Autodesk Inventor part; units mm, degrees
(part 2 of 2)
sketch "Sketch70" plane through (80, 0, -85) normal (-1, 0, 0) x (0, 0, 1)
  line L0 (155.5, 281.1154) -> (155.5, 497.1154) projected
  line L1 (155.5, 497.1154) -> (14.5, 497.1154) projected
  line L2 (14.5, 497.1154) -> (14.5, 281.1154) projected
  line L3 (14.5, 281.1154) -> (155.5, 281.1154) projected
  line L4 (155.5, 281.1154) -> (14.5, 281.1154) projected
  point P0 (85, 0)
  point P1 (150.5, 492.1154)
  point P2 (105.5, 492.1154)
  point P3 (150.5, 452.1154)
  point P4 (150.5, 412.1154)
  point P5 (150.5, 286.1154)
  point P6 (19.5, 492.1154)
  point P7 (64.5, 492.1154)
  point P8 (19.5, 452.1154)
  point P9 (19.5, 412.1154)
  point P10 (19.5, 286.1154)
  point P11 (64.5, 286.1154)
  point P12 (105.5, 286.1154)
  point P13 (19.5, 326.1154)
  point P14 (19.5, 366.1154)
  point P15 (150.5, 326.1154)
  point P16 (150.5, 366.1154)
  dimension "d780" = 5
  dimension "d781" = 5
  dimension "d784" = 45
  dimension "d791" = 40
  dimension "d796" = 5
  dimension "d797" = 5
  dimension "d800" = 45
  dimension "d807" = 40
  dimension "d814" = 45
  dimension "d821" = 45
  dimension "d826" = 5
  dimension "d827" = 5
  dimension "d828" = 5
  dimension "d829" = 5
  dimension "d832" = 40
  dimension "d839" = 40
  constraints: 4 horizontal, 4 vertical, 12 other
  measures "d780" distance from line of point (150.5, 492.115) L0
  measures "d781" distance from line of L1 point (150.5, 492.115)
  measures "d784" distance of point (150.5, 492.115) point (105.5, 492.115)
  measures "d791" distance of point (150.5, 492.115) point (150.5, 452.115)
  measures "d796" distance from line of L2 point (19.5, 492.115)
  measures "d797" distance from line of L1 point (19.5, 492.115)
  measures "d800" distance of point (19.5, 492.115) point (64.5, 492.115)
  measures "d807" distance of point (19.5, 492.115) point (19.5, 452.115)
  measures "d814" distance of point (19.5, 286.115) point (64.5, 286.115)
  measures "d821" distance of point (150.5, 286.115) point (105.5, 286.115)
  measures "d826" distance from line of L4 point (19.5, 286.115)
  measures "d827" distance from line of L2 point (19.5, 286.115)
  measures "d828" distance from line of L3 point (150.5, 286.115)
  measures "d829" distance from line of point (150.5, 286.115) L0
  measures "d832" distance of point (19.5, 286.115) point (19.5, 326.115)
  measures "d839" distance of point (150.5, 286.115) point (150.5, 326.115)
hole "Hole32" at (80, 492.1154, 65.5) at (80, 492.1154, 20.5) at (80, 452.1154, 65.5) at (80, 412.1154, 65.5) at (80, 286.1154, 65.5) at (80, 492.1154, -65.5) at (80, 492.1154, -20.5) at (80, 452.1154, -65.5) at (80, 412.1154, -65.5) at (80, 286.1154, -65.5) at (80, 286.1154, -20.5) at (80, 286.1154, 20.5) at (80, 326.1154, -65.5) at (80, 366.1154, -65.5) at (80, 326.1154, 65.5) at (80, 366.1154, 65.5) direction (1, 0, 0) diameter 2.459 depth 5 tip angle 118 bodies 13
body "Solid3"
body "Solid12"
body "Solid25"
body "Solid26"
body "Solid27"
body "Solid29"
body "Solid18"
body "Solid19"
body "Solid20"
body "Solid23"
